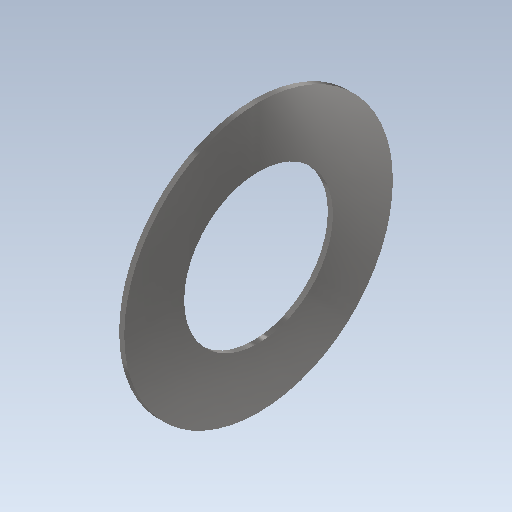
# Autodesk Inventor part: F606ZZ Shield2
Saved by Autodesk Inventor 2020.3 (Build 243373000, 373)
## iProperties
Part Number: F606ZZ Shield2
Material: 鋼、炭素鋼
Catalog Web Link: www.cadenas.de
Description: shielded_type_zz_zzs_S2-
Vendor: NSK_RB
Document SubType Name: Modeling
Designer: partserver
Manufacturer: NSK_RB
Mass: 0.263083 g
Surface Area: 2.58758 cm^2
Volume: 0.0335137 cm^3
Density: 7.85 g/cm^3
Appearance: 半つや出し
Category: PARTsolutions
Company: NSK_RB
PSOL_IDENT_0: {$CADENAS_DATA\23d-libs\nsk_rb\roller_bearings\deep_groove_bb\exstra_small_miniatur_bb\metric_design
PSOL_IDENT_1: _with_flange\shielded_type_zz_zzs_s2_1.prj},186 {VTYP=3D},{NB=F606ZZ Shield2},{LINA=F606ZZ Shield2},
PSOL_IDENT_2: {NN=shielded_type_zz_zzs_S2},{DATE=10.04.2020 04:57:40},{GEOMDATE=04.01.2008 00:00:00},{VERSION=},{L
PSOL_IDENT_3: INEID=540},{WBVAR=},{WBNUMERIC=}  {NB=F606ZZ Shield2},{LINA=F606ZZ Shield2},{KT=DUMMY},{IDNR=},{STAN=
PSOL_IDENT_4: },{ORDER=F606ZZ},{SD=6.0},{X=6.0},{D=17},{DD=17},{DD1=0.0},{D2=19.0},{DD2=19.0},{B=0.0},{B1=6.0},{CC
PSOL_IDENT_5: 1=0.0},{C2=1.2},{CC2=1.2},{R=0.00},{R1=0.30},{DI1=8.92},{DI2=8.20},{SDE1=13.75},{SDE2=14.80},{CR1=22
PSOL_IDENT_6: 60},{COR1=835},{CR2=231},{COR2=85.0},{LG=38000},{LO=45000},{DA=0.0},{DB=8.2},{RA=0.00},{RB=0.30},{MA
PSOL_IDENT_7: SS=6.61},{SC=1}
NB: F606ZZ Shield2
NN: shielded_type_zz_zzs_S2
NBSYN: $ORDER. Shield2
LINA: F606ZZ Shield2
CATALOG: NSK Rolling Bearing
ORDER: F606ZZ
SD: 6
X: 6
D: 17
DD: 17
DD1: 0
D2: 19
DD2: 19
B: 0
B1: 6
CC1: 0
C2: 1.2
CC2: 1.2
R: 0
R1: 0.3
DI1: 8.92
DI2: 8.2
SDE1: 13.75
SDE2: 14.8
CR1: 2260
COR1: 835
CR2: 231
COR2: 85
LG: 38000
LO: 45000
DA: 0
DB: 8.2
RA: 0
RB: 0.3
MASS: 6.61
SC: 1
SUPPLIER: NSK_RB
ARTICLENO: F606ZZ Shield2
BOMINFO: F606ZZ Shield2
CREATOR: CADENAS GmbH
Title: F606ZZ Shield2
Author: Cadenas PARTsolutions
Autodesk Inventor part; units mm, degrees
sketch "Sketch_1" plane through (0, 0, 0) normal (0, 0, 1) x (1, 0, 0)
  line L0 (5.9061, 0) -> (5.625, 0)
  line L1 (5.625, 4.1) -> (5.9061, 4.1)
  line L2 (5.9061, 4.1) -> (5.9061, 7.4)
  line L3 (5.9061, 7.4) -> (5.625, 7.4)
  line L4 (5.625, 7.4) -> (5.625, 4.1)
  constraints: 10 end point
revolve "Revolution1" add sketch "Sketch_1" angle 360 about axis through (5.9061, 0, 0) along (1, 0, 0)
ref_plane "ip_st_1_XY" through (5.625, 0, 0) normal (1, 0, 0) x (0, 0, -1)
ref_plane "ip_st_1_YZ" through (5.625, 0, 0) normal (0, 0, -1) x (0, 1, 0)
ref_plane "ip_st_1_ZX" through (5.625, 0, 0) normal (0, 1, 0) x (1, 0, 0)
body "Solid1"
